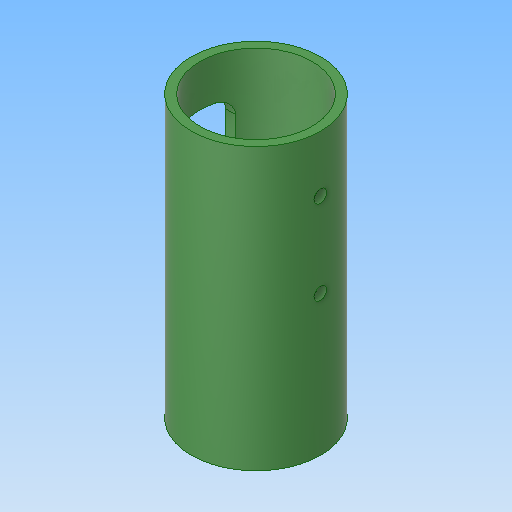
# Autodesk Inventor part: Pancake_PVC Pipe
Saved by Autodesk Inventor 2018.1 (Build 221171000, 171)
## iProperties
Created: 2019-02-11
Part Number: Pancake_PVC Pipe
Material: PVC-Piping
Document SubType Name: Modeling
Designer: James
Density: 1.4 g/cm^3
Appearance: Smooth - Dark Forest Green
Mass: 50.1487 g
Surface Area: 253.785 cm^2
Volume: 35.8205 cm^3
Author: James
Autodesk Inventor part; units mm, degrees
ref_plane "YZ Plane" through (0, 0, 0) normal (1, 0, 0) x (0, 1, 0)
ref_plane "XZ Plane" through (0, 0, 0) normal (0, 1, 0) x (-1, 0, 0)
ref_plane "XY Plane" through (0, 0, 0) normal (0, 0, 1) x (1, 0, 0)
sketch "Sketch1" plane through (0, 0, 0) normal (0, 1, 0) x (-1, 0, 0)
  circle A0 centre (0, 0) radius 23
  circle A1 centre (0, 0) radius 20
  dimension "d0" = 3
  dimension "d1" = 40
  constraints: 2 centre point, 2 coincident
  measures "d0" radial gap between concentric circles of A0 A1
  measures "d1" diameter of A1
extrude "Extrusion1" add sketch "Sketch1" along normal blind 100
sketch "Sketch2" plane through (0, 0, 0) normal (0, 0, 1) x (1, 0, 0)
  line L0 (-23, 85) -> (0, 85)
  line L1 (0, 85) -> (0, 10)
  line L2 (0, 10) -> (-23, 10)
  line L3 (-23, 10) -> (-23, 85)
  line L4 (23, 100) -> (-23, 100) projected
  line L5 (-23, 0) -> (23, 0) projected
  point P0 (0, 0)
  dimension "d4" = 75
  dimension "d5" = 10
  constraints: 8 end point, 2 parallel, 1 horizontal, 1 perpendicular, 1 vertical alignment
  measures "d4" distance of L2.end L0.start
  measures "d5" distance between parallel lines of L5 L2
extrude "Extrusion2" cut sketch "Sketch2" along normal mid plane 20
fillet "Fillet1" radius 5 4 edges at (-19.0164, 85, -10) (-19.0164, 85, 10) (-19.0164, 10, 10) (-19.0164, 10, -10)
sketch "Sketch3" plane through (0, 0, 0) normal (1, 0, 0) x (0, 1, 0)
  line L0 (-20, 0) -> (120, 0) projected
  line L1 (85, -5) -> (85, 5) projected
  line L2 (100, 20) -> (100, -20) projected
  point P0 (0, 0)
  point P1 (80, 0)
  point P2 (50, 0)
  dimension "d9" = 30
  dimension "d18" = 20
  constraints: 1 horizontal alignment, 1 point on line
  measures "d9" distance of point (50, 0) point (80, 0)
  measures "d18" distance from line of L2 point (80, 0)
hole "Hole1" at (0, 80, 0) at (0, 50, 0) direction (1, 0, 0) diameter 4.5 end through all clearance for "Socket Head Cap Screw" size "M4" standard "Ansi Metric M Profile"
body "Solid1"
